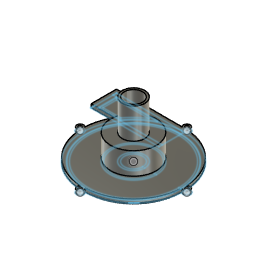
Top v2 (Autodesk Fusion 360 design; units mm, degrees)
Autodesk Fusion 360 part; units mm, degrees
note: some values were not read from the file. Set by a fixed rule: which sketch regions a step uses.
sketch "Skizze1" plane through (0, 0, 0) normal (0, 0, 1) x (1, 0, 0)
  line L0 (-40, 17) -> (0, 17)
  line L1 (0, 30) -> (-40, 30)
  line L2 (-40, 15) -> (0, 15)
  circle A0 centre (0, 31.5) radius 2
  line L3 (-40, 28) -> (0, 28)
  circle A1 centre (0, 0) radius 30
  circle A2 centre (0, 31.5) radius 1
  line L4 (0, 15) -> (0, 30)
  line L5 (-40, 15) -> (-40, 17)
  line L6 (-40, 30) -> (-40, 15)
  circle A3 centre (-31.5, 0) radius 1
  circle A4 centre (0, -31.5) radius 2
  circle A5 centre (31.5, 0) radius 2
  circle A6 centre (31.5, 0) radius 1
  circle A7 centre (0, 0) radius 28
  circle A8 centre (0, -31.5) radius 1
  line L7 (-40, 30) -> (-40, 28)
  circle A9 centre (-31.5, 0) radius 2
  line L8 (-38, 28) -> (-38, 17)
  line L9 (-38, 27.5) -> (-37.5, 27.5)
  line L10 (-37.5, 27.5) -> (-37.5, 17.5)
  line L11 (-37.5, 17.5) -> (-25, 17.5)
  line L12 (-37.5, 27.5) -> (-13.5, 27.5)
  arc A10 (-13.5, 27.5) -> (-25, 17.5) centre (0.0202, 0.3392) ccw
  line L13 (-36.5, 26.5) -> (-17.5, 26.5)
  line L14 (-36.5, 26.5) -> (-36.5, 18.5)
  line L15 (-36.5, 18.5) -> (-26, 18.5)
  arc A11 (-17.5, 26.5) -> (-26, 18.5) centre (-0.9044, 0.3515) ccw
  circle A12 centre (0, 0) radius 27.75
  circle A13 centre (0, 0) radius 26.75
  circle A14 centre (0, 0) radius 6.625
  circle A15 centre (0, 0) radius 5.375
  circle A16 centre (0, 0) radius 12.5
  circle A17 centre (0, 0) radius 13.5
  dimension "d1" = 60
  dimension "d7" = 2
  dimension "d8" = 4
  dimension "d9" = 2
  dimension "d10" = 4
  dimension "d11" = 2
  dimension "d12" = 4
  dimension "d13" = 2
  dimension "d14" = 4
  dimension "d15" = 40
  dimension "d16" = 15
  dimension "d17" = 2
  dimension "d18" = 56
  dimension "d19" = 2
  dimension "d20" = 0.5
  dimension "d21" = 55.5
  dimension "d22" = 53.5
  dimension "d29" = 13.25
  dimension "d30" = 10.75
  dimension "d39" = 25
  dimension "d40" = 27
  constraint coincident A1.centre A7.centre
  constraint concentric A3 A9
  constraint concentric A5 A6
  constraint concentric A4 A8
  constraint concentric A0 A2
  constraint horizontal L1
  constraint vertical L6
  constraint horizontal L2
  constraint vertical L4
  constraint coincident L1.start A1
  constraint perpendicular L1 L7
  constraint coincident L3.end L4
  constraint perpendicular L3 L4
  constraint perpendicular L2 L5
  constraint coincident L0.end L4
  constraint perpendicular L0 L4
  constraint coincident L8.start L3
  constraint coincident L8.end L0
  constraint perpendicular L0 L8
  constraint coincident L8 L9.start
  constraint perpendicular L8 L9
  constraint perpendicular L0 L10
  constraint perpendicular L10 L11
  constraint perpendicular L10 L12
  constraint tangent A1 A10
  constraint perpendicular L10 L13
  constraint perpendicular L13 L14
  constraint perpendicular L14 L15
  constraint tangent A1 A11
  constraint concentric A7 A12
  constraint concentric A7 A13
  constraint concentric A13 A14
  constraint concentric A12 A15
  constraint concentric A14 A16
  constraint concentric A14 A17
  measures "d1" diameter of A1
  measures "d7" diameter of A3
  measures "d8" diameter of A9
  measures "d9" diameter of A6
  measures "d10" diameter of A5
  measures "d11" diameter of A8
  measures "d12" diameter of A4
  measures "d13" diameter of A2
  measures "d14" diameter of A0
  measures "d15" distance of L1.end L1.start
  measures "d16" distance of L1.start L2.end
  measures "d17" distance of L1.end L3.start
  measures "d18" diameter of A7
  measures "d19" distance of L2.start L0.start
  measures "d20" distance of L9.start L9.end
  measures "d21" diameter of A12
  measures "d22" diameter of A13
  measures "d29" diameter of A14
  measures "d30" diameter of A15
  measures "d39" diameter of A16
  measures "d40" diameter of A17
extrude "Extrusion3" add sketch "Skizze1" along normal blind 2 contours L0 L3 L6 L8 | L0 L2 A1 L5 L6 | L0 L3 A1 L8 | L1 A0 L3 A1 L6 L7 | L0 L3 A1 A7 | L0 L2 A1 A7 | L2 A0 A1 L4 A4 A5 A7 A9 | L0 L4 A7 A12 | L0 L2 A7 A12 | A0 L3 A1 L4 | L2 L4 A7 A12 | A1 A9 | A1 A9 | L1 A0 A1 | L1 A0 A1 | A0 A1 L4 | A0 A1 L4 | L0 L4 A13 | L0 L2 L4 A13 | L2 L4 A13 | A1 A4 | A1 A4 | A1 A5 | A1 A5 | L13 L14 L15 A11 makes body 1 at (-33, 21.1667, 0) makes body 2 at (-39.1667, 24.1667, 0) makes body 3 at (22.1835, -1.9997, 0)
extrude "Extrusion4" add sketch "Skizze1" along normal blind 2 and the other way blind 2 contours L0 L4 A12 A13 | L0 L2 A12 A13 | L2 L4 A12 A13 | L10 L11 L12 A10 bodies 1 2 3
extrude "Extrusion6" add sketch "Skizze1" along normal blind 15 contours A17 bodies 1
extrude "Extrusion7" add sketch "Skizze1" along normal blind 2 from surface at 13 contours A16 bodies 1
extrude "Extrusion8" add sketch "Skizze1" along normal blind 20 from surface at 13 contours A14 bodies 1
